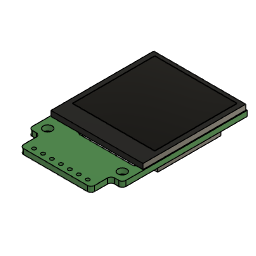
PicoDesktopPenHolder-v10 (Autodesk Fusion 360 archive; units mm, degrees)
design "LCD Square 1.3 SPI"
Autodesk Fusion 360 part; units mm, degrees
sketch "PCB" plane through (0, 0, 0) normal (0, 0, 1) x (1, 0, 0) in component "Board"
  line L0 (0, 13.01) -> (-13.3, 13.01)
  line L1 (-13.3, 13.01) -> (-13.3, -21.53)
  line L2 (-12.3, -22.53) -> (-11.1, -22.53)
  line L3 (-10.1, -23.53) -> (-10.1, -27.23)
  line L4 (-9.1, -28.23) -> (0, -28.23)
  line L5 (0, 19) -> (0, -24)
  line L6 (0, 13.01) -> (13.3, 13.01)
  line L7 (13.3, 13.01) -> (13.3, -22.53)
  line L8 (10.1, -22.53) -> (10.1, -28.23)
  line L9 (-15, -19.83) -> (15, -19.83) construction
  circle A0 centre (-10.6, -19.83) radius 1.25
  circle A1 centre (10.6, -19.83) radius 1.25
  line L10 (-11, -26.73) -> (11, -26.73) construction
  circle A2 centre (-7.6, -26.73) radius 0.5
  circle A3 centre (-5.0533, -26.73) radius 0.5
  circle A4 centre (-2.5067, -26.73) radius 0.5
  circle A5 centre (0.04, -26.73) radius 0.5
  circle A6 centre (2.5867, -26.73) radius 0.5
  circle A7 centre (5.1333, -26.73) radius 0.5
  circle A8 centre (7.68, -26.73) radius 0.5
  line L11 (-4.5, -5.8) -> (10.5, -5.8)
  line L12 (11.5, -6.8) -> (11.5, -15.8)
  line L13 (10.5, -16.8) -> (-4.5, -16.8)
  line L14 (-5.5, -15.8) -> (-5.5, -6.8)
  arc A9 (-4.5, -5.8) -> (-5.5, -6.8) centre (-4.5, -6.8) ccw
  arc A10 (11.5, -6.8) -> (10.5, -5.8) centre (10.5, -6.8) ccw
  arc A11 (-5.5, -15.8) -> (-4.5, -16.8) centre (-4.5, -15.8) ccw
  arc A12 (10.5, -16.8) -> (11.5, -15.8) centre (10.5, -15.8) ccw
  arc A13 (-13.3, -21.53) -> (-12.3, -22.53) centre (-12.3, -21.53) ccw
  arc A14 (-10.1, -23.53) -> (-11.1, -22.53) centre (-11.1, -23.53) ccw
  arc A15 (-10.1, -27.23) -> (-9.1, -28.23) centre (-9.1, -27.23) ccw
  arc A16 (9.1, -28.23) -> (10.1, -27.23) centre (9.1, -27.23) ccw
  arc A17 (11.1, -22.53) -> (10.1, -23.53) centre (11.1, -23.53) ccw
  arc A18 (12.3, -22.53) -> (13.3, -21.53) centre (12.3, -21.53) ccw
  line L15 (12.3, -22.53) -> (11.1, -22.53)
  line L16 (9.1, -28.23) -> (0, -28.23)
  point P0 (-10.1, -28.23)
  point P1 (-5.5, -5.8)
  point P2 (11.5, -16.8)
  point P3 (-5.5, -16.8)
  dimension "d1" = 13.01
  dimension "d2" = 26.6
  dimension "d3" = 41.24
  dimension "d4" = 8.4
  dimension "d5" = 5.7
  dimension "d6" = 20.2
  dimension "d7" = 13.3
  dimension "d8" = 2.5
  dimension "d9" = 21.2
  dimension "d10" = 1.5
  dimension "d11" = 1
  dimension "d12" = 2.5
  dimension "d15" = 15.28
  dimension "d16" = 0
  dimension "d17" = 2.5467
  dimension "d18" = 5.5
  dimension "d19" = 17
  dimension "d20" = 5.8
  dimension "d21" = 11
  dimension "d22" = 1
  dimension "d23" = 1
  dimension "d24" = 1
  dimension "d25" = 1
  dimension "d26" = 1
  dimension "d27" = 1
  dimension "d28" = 1
  constraint horizontal L0
  constraint perpendicular L0 L1
  constraint perpendicular L1 L2
  constraint perpendicular L2 L3
  constraint perpendicular L3 L4
  constraint perpendicular L4 L5
  constraint symmetric L0.start L5 L6.start
  constraint symmetric L0.end L5 L6.end
  constraint symmetric P0 L5 L8.end
  constraint perpendicular L7 L9
  constraint coincident L9 A0.centre
  constraint symmetric L5 A0 A1
  constraint perpendicular L8 L10
  constraint coincident L10 A2.centre
  constraint horizontal L11
  constraint vertical L12
  constraint horizontal L13
  constraint vertical L14
  constraint coincident P1 L14
  constraint coincident P1 L11
  constraint tangent L14 A9
  constraint tangent L11 A9
  constraint tangent L11 A10
  constraint tangent L12 A10
  constraint coincident P3 L14
  constraint coincident P3 L13
  constraint tangent L14 A11
  constraint tangent L13 A11
  constraint coincident P2 L13
  constraint coincident P2 L12
  constraint tangent L13 A12
  constraint tangent L12 A12
  constraint tangent L1 A13
  constraint tangent L2 A13
  constraint tangent L2 A14
  constraint tangent L3 A14
  constraint coincident P0 L3
  constraint coincident P0 L4
  constraint tangent L3 A15
  constraint tangent L4 A15
  constraint symmetric L5 L3.end A16.end
  constraint symmetric L5 L4.start A16.start
  constraint symmetric L5 A15 A16
  constraint symmetric L5 L2.end A17.start
  constraint symmetric L5 L3.start A17.end
  constraint symmetric L5 A14 A17
  constraint symmetric L5 L1.end A18.end
  constraint symmetric L5 L2.start A18.start
  constraint symmetric L5 A13 A18
  constraint symmetric L4.end L5 L16.end
  measures "d1" distance of origin L0
  measures "d2" distance of L1 L7
  measures "d3" distance of L0 L4
  measures "d4" distance of L4 L9
  measures "d5" distance of L2 P0
  measures "d6" distance of L3 L8
  measures "d7" distance of origin L1
  measures "d8" diameter of A0
  measures "d9" distance of A0.centre A1.centre
  measures "d10" distance of L4 L10
  measures "d11" diameter of A2
  measures "d12" distance of L3 A2.centre
  measures "d17" distance of A2.centre A3.centre
  measures "d18" distance of origin L14
  measures "d19" distance of P2 P3
  measures "d20" distance of origin L11
  measures "d21" distance of P1 P3
  measures "d22" radius of A9
  measures "d23" radius of A10
  measures "d24" radius of A11
  measures "d25" radius of A12
  measures "d26" radius of A13
  measures "d27" radius of A14
  measures "d28" radius of A15
extrude "Extrude1" add sketch "PCB" along normal blind 1.5 makes body 1 in component "Board"
sketch "Display" plane through (0, 0, 0) normal (0, 0, 1) x (1, 0, 0) in component "Display"
  line L0 (-13.08, 12.79) -> (13.08, 12.79)
  line L1 (13.08, 12.79) -> (13.08, -16.43)
  line L2 (13.08, -16.43) -> (-13.08, -16.43)
  line L3 (-13.08, -16.43) -> (-13.08, 12.79)
  line L4 (0, 0) -> (0, 16)
  line L5 (-11.7, 11.7) -> (11.7, 11.7)
  line L6 (11.7, 11.7) -> (11.7, -11.7)
  line L7 (11.7, -11.7) -> (-11.7, -11.7)
  line L8 (-11.7, -11.7) -> (-11.7, 11.7)
  line L9 (0, 0) -> (25, 0) construction
  arc A0 (-5.5, -15.8) -> (-4.5, -16.8) centre (-4.5, -15.8) ccw construction
  line L10 (-5.5, -15.8) -> (-5.5, -6.8) construction
  arc A1 (-4.5, -5.8) -> (-5.5, -6.8) centre (-4.5, -6.8) ccw construction
  line L11 (-4.5, -5.8) -> (10.5, -5.8) construction
  arc A2 (11.5, -6.8) -> (10.5, -5.8) centre (10.5, -6.8) ccw construction
  line L12 (11.5, -6.8) -> (11.5, -15.8) construction
  arc A3 (10.5, -16.8) -> (11.5, -15.8) centre (10.5, -15.8) ccw construction
  line L13 (10.5, -16.8) -> (-4.5, -16.8) construction
  circle A4 centre (-10.6, -19.83) radius 1.25 construction
  circle A5 centre (7.68, -26.73) radius 0.5 construction
  circle A6 centre (-5.0533, -26.73) radius 0.5 construction
  circle A7 centre (5.1333, -26.73) radius 0.5 construction
  circle A8 centre (-7.6, -26.73) radius 0.5 construction
  circle A9 centre (-2.5067, -26.73) radius 0.5 construction
  circle A10 centre (0.04, -26.73) radius 0.5 construction
  circle A11 centre (2.5867, -26.73) radius 0.5 construction
  circle A12 centre (10.6, -19.83) radius 1.25 construction
  arc A13 (12.3, -22.53) -> (13.3, -21.53) centre (12.3, -21.53) ccw construction
  line L14 (13.3, -21.53) -> (13.3, 13.01) construction
  line L15 (13.3, 13.01) -> (-13.3, 13.01) construction
  line L16 (-13.3, 13.01) -> (-13.3, -21.53) construction
  arc A14 (-13.3, -21.53) -> (-12.3, -22.53) centre (-12.3, -21.53) ccw construction
  line L17 (-12.3, -22.53) -> (-11.1, -22.53) construction
  arc A15 (-10.1, -23.53) -> (-11.1, -22.53) centre (-11.1, -23.53) ccw construction
  line L18 (-10.1, -23.53) -> (-10.1, -27.23) construction
  arc A16 (-10.1, -27.23) -> (-9.1, -28.23) centre (-9.1, -27.23) ccw construction
  line L19 (-9.1, -28.23) -> (9.1, -28.23) construction
  arc A17 (9.1, -28.23) -> (10.1, -27.23) centre (9.1, -27.23) ccw construction
  line L20 (10.1, -27.23) -> (10.1, -23.53) construction
  arc A18 (11.1, -22.53) -> (10.1, -23.53) centre (11.1, -23.53) ccw construction
  line L21 (11.1, -22.53) -> (12.3, -22.53) construction
  dimension "d31" = 26.16
  dimension "d32" = 29.22
  dimension "d33" = 23.4
  dimension "d34" = 23.4
  dimension "d36" = 11.8
  constraint horizontal L0
  constraint vertical L1
  constraint horizontal L2
  constraint vertical L3
  constraint coincident L4.start L9.start
  constraint perpendicular L0 L4
  constraint symmetric L1 L3 L4
  constraint horizontal L5
  constraint vertical L6
  constraint horizontal L7
  constraint vertical L8
  constraint symmetric L4 L6 L8
  constraint perpendicular L6 L9
  constraint symmetric L5 L7 L9
  measures "d31" distance of L0.start L0.end
  measures "d32" distance of L0.start L2.end
  measures "d33" distance of L5.start L5.end
  measures "d34" distance of L5.start L7.end
  measures "d36" distance of L2 L19
extrude "Extrude1'" add sketch "Display" along normal blind 1.5 from surface at 1.5 separate body contours L0 L1 L2 L3 | L5 L6 L7 L8 makes body 2 in component "Display"
extrude "Extrude2" add sketch "Display" along normal blind 0.1 from surface at 3 contours L5 L6 L7 L8 bodies 2 in component "Display"
sketch "Components" plane through (0, 0, 0) normal (0, 0, 1) x (1, 0, 0) in component "Components"
  line L0 (-12.8, 6.01) -> (12.8, 6.01)
  line L1 (12.8, 6.01) -> (12.8, -11.99)
  line L2 (12.8, -11.99) -> (-12.8, -11.99)
  line L3 (-12.8, -11.99) -> (-12.8, 6.01)
  line L4 (-13.3, 13.01) -> (-13.3, -21.53)
  line L5 (13.3, -21.53) -> (13.3, 13.01)
  line L6 (13.3, 13.01) -> (-13.3, 13.01)
  dimension "d43" = 7
  dimension "d44" = 18
  dimension "d45" = 0.5
  dimension "d46" = 0.5
  constraint horizontal L0
  constraint vertical L1
  constraint horizontal L2
  constraint vertical L3
  measures "d43" distance of L0 L6
  measures "d44" distance of L0.start L2.end
  measures "d45" distance of L3 L4
  measures "d46" distance of L1 L5
extrude "Extrude1''" add sketch "Components" against normal blind 1.5 separate body makes body 3 in component "Components"
component "Board" placed x (1, 0, 0) y (0, 1, 0) z (0, 0, 1) at (0, 0, 0)
component "Display" placed x (1, 0, 0) y (0, 1, 0) z (0, 0, 1) at (0, 0, 0)
component "Components" placed x (1, 0, 0) y (0, 1, 0) z (0, 0, 1) at (0, 0, 0)
named bodies: "PCB", "Display box", "Components"
